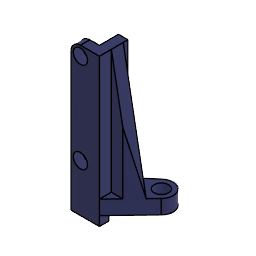
ServoDriverBracket_v12 (Autodesk Fusion 360 design; units mm, degrees)
Autodesk Fusion 360 part; units mm, degrees
sketch "Sketch1" plane through (0, 0, 0) normal (0, 1, 0) x (1, 0, 0)
  line L0 (0, 0) -> (0, -19) construction
  circle A0 centre (0, -19) radius 1.5
  circle A1 centre (0, 0) radius 1.5
  line L1 (2, 2) -> (-2, 2)
  line L2 (-2, 2) -> (-2, -21)
  line L3 (-2, -21) -> (2, -21)
  line L4 (2, -21) -> (2, 2)
  line L5 (2, 2) -> (-2, -21) construction
  line L6 (-2, 2) -> (2, -21) construction
  line L7 (2, -21) -> (4, -21)
  line L8 (4, -21) -> (4, 2)
  line L9 (4, 2) -> (2, 2)
  line L10 (2, 2) -> (2, -21)
  point P0 (0, -9.5)
  dimension "d1" = 19
  dimension "d2" = 3
  dimension "d3" = 3
  dimension "d4" = 2
  dimension "d5" = 2
  constraint coincident L0.start A1.centre
  constraint vertical L0
  constraint coincident L0.end A0.centre
  constraint horizontal L1
  constraint perpendicular L1 L2
  constraint parallel L1 L3
  constraint parallel L2 L4
  constraint coincident L5 P0
  constraint coincident L6 P0
  constraint midpoint L0 P0
  constraint horizontal L7
  constraint vertical L8
  constraint horizontal L9
  constraint vertical L10
  measures "d1" distance of L0.start L0.end
  measures "d2" diameter of A0
  measures "d3" diameter of A1
  measures "d4" distance of L0.end L3
  measures "d5" distance of L0.end L4
extrude "Extrude1" add sketch "Sketch1" along normal blind 2
fillet "Fillet1" radius 2 1 edges at (-2, 1, 21)
extrude "Extrude2" add sketch "Sketch1" along normal blind 6 contours L4 L7 L8 L9 L10
move_face "OffsetFaces1" offset 3 1 faces at (3.3333, 2.6667, -2)
sketch "Sketch2" plane through (0, 0, -5) normal (0, 0, -1) x (1, 0, 0)
  line L0 (4, 0) -> (-2, 0)
  line L1 (-2, 0) -> (-2, -2)
  line L2 (-2, -2) -> (2, -2)
  line L3 (2, -2) -> (2, -6)
  line L4 (2, -6) -> (4, -6)
  line L5 (4, -6) -> (4, 0)
  line L6 (4, -6) -> (8.6195, -8.3843) construction
  circle A0 centre (8.6195, -8.3843) radius 2.5
  circle A1 centre (8.6195, -8.3843) radius 1.5
  line L7 (2, -6) -> (6.9918, -10.2818)
  line L8 (10.4671, -6.7002) -> (4, 0)
  circle A2 centre (8.6195, -8.3843) radius 3 construction
  line L9 (4, -5) -> (8.8261, -5)
  line L10 (4, -2.5) -> (6.413, -2.5)
  dimension "d12" = 5
  dimension "d13" = 3
  dimension "d19" = 6
  constraint coincident L4.end L5.start
  constraint coincident L6.end A0.centre
  constraint concentric A0 A1
  constraint coincident L3.end L4.start
  constraint coincident A0 L7.end
  constraint tangent A0 L7
  constraint coincident A0 L8.start
  constraint coincident L0.start L5.end
  constraint concentric A0 A2
  constraint coincident L5 L9.start
  constraint coincident L8 L9.end
  constraint perpendicular L5 L9
  constraint coincident L5 L10.start
  constraint coincident L8 L10.end
  constraint perpendicular L5 L10
  measures "d12" diameter of A0
  measures "d13" diameter of A1
  measures "d19" diameter of A2
extrude "Extrude3" add sketch "Sketch2" along normal blind 3
sketch "Sketch3" plane through (0, 0, -8) normal (0, 0, -1) x (1, 0, 0)
  circle A0 centre (8.6195, -8.3843) radius 1.5
  line L0 (2, -6) -> (6.9918, -10.2818)
  arc A1 (6.9918, -10.2818) -> (10.3679, -6.5974) centre (8.6195, -8.3843) ccw
  line L1 (10.3679, -6.5974) -> (4, 0)
  line L2 (4, 0) -> (-2, 0)
  line L3 (-2, 0) -> (-2, -2)
  line L4 (-2, -2) -> (2, -2)
  line L5 (2, -2) -> (2, -6)
  line L6 (4, 0) -> (4, -2)
  line L7 (4, -2) -> (2, -2)
  constraint coincident L1.end L2.start
  constraint perpendicular L2 L6
  constraint coincident L4.end L5.start
extrude "Extrude4" add sketch "Sketch3" along normal blind 2 contours L2 L3 L4 L6 L7
extrude "Extrude5" add sketch "Sketch2" against normal blind 28.3 contours L5 L8 L9 L10
sketch "Sketch4" plane through (0, 5, 0) normal (0, 1, 0) x (-1, 0, 0)
  line L0 (-8.8261, -5) -> (-4, -5)
  line L1 (-4, -5) -> (-4, 21)
  line L2 (-4, 23.3) -> (-8.8261, 23.3)
  line L3 (-8.8261, 23.3) -> (-8.8261, -5)
  line L4 (-4, 21) -> (-8.8261, -5)
  line L5 (-4, 21) -> (-4, 23.3)
  constraint coincident L1.end L4.start
  constraint coincident L0.start L3.end
extrude "Extrude6" cut sketch "Sketch4" against normal blind 15 contours L2 L3 L4 L5
delete_face "DeleteFace1" 1 faces at (3.3333, 2, -8.6667)
